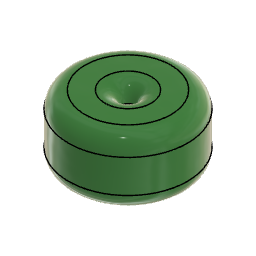
Puck_10 mm h v1 (Autodesk Fusion 360 design; units mm, degrees)
Autodesk Fusion 360 part; units mm, degrees
sketch "Sketch1" plane through (0, 0, 0) normal (0, 0, 1) x (1, 0, 0)
  circle A0 centre (25, 25) radius 9
  circle A1 centre (25, 25) radius 1
  dimension "d1" = 18
  dimension "d2" = 2
  constraint concentric A0 A1
  measures "d1" diameter of A0
  measures "d2" diameter of A1
extrude "Extrude1" add sketch "Sketch1" along normal blind 10
fillet "Fillet1" radius 2.5 4 faces at (31.2961, 24.5032, 10) (25.7971, 25.6038, 6.6667) (33.9888, 24.5514, 6.6667) (31.2961, 24.5032, 0)
